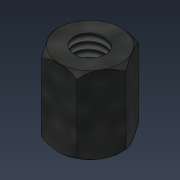
# Autodesk Inventor part: M2.5x5
Saved by Autodesk Inventor 2022.1 (Build 261234020, 234B)
## iProperties
Created: 2012-08-14
Part Number: M2.5x5
Material: Stahl
Document SubType Name: Modeling
Designer: rYan
Density: 7.85 g/cm^3
Mass: 3.36246 g
Surface Area: 5.74911 cm^2
Volume: 0.428339 cm^3
Appearance: Platte
Author: rYan
Autodesk Inventor part; units mm, degrees
ref_plane "YZ Plane" through (0, 0, 0) normal (1, 0, 0) x (0, 1, 0)
ref_plane "XZ Plane" through (0, 0, 0) normal (0, 1, 0) x (-1, 0, 0)
ref_plane "XY Plane" through (0, 0, 0) normal (0, 0, 1) x (1, 0, 0)
sketch "Skizze1" plane through (0, 0, 0) normal (0, 0, 1) x (1, 0, 0)
  line L0 (2.3094, 0) -> (1.1547, -2)
  line L1 (1.1547, -2) -> (-1.1547, -2)
  line L2 (-1.1547, -2) -> (-2.3094, 0)
  line L3 (-2.3094, 0) -> (-1.1547, 2)
  line L4 (-1.1547, 2) -> (1.1547, 2)
  line L5 (1.1547, 2) -> (2.3094, 0)
  point P0 (0, 0)
  point P1 (0, 0)
  dimension "SW" = 4
  constraints: 12 end point, 1 coincident, 13 other
  measures "SW" distance between parallel lines of L1 L4
extrude "Extrusion1" add sketch "Skizze1" along normal mid plane 5
sketch "Skizze2" plane through (0, 0, 2.5) normal (0, 0, 1) x (1, 0, 0)
  point P0 (0, 0)
  point P1 (0, 0)
  constraints: 1 coincident
hole "Bohrung1" at (0, 0, 2.5) direction (0, 0, -1) diameter 2.013 end through all thread size "M2.5x0.45" class "6H" standard "ISO Metric profile"
sketch "Innenradius" plane through (0, 0, 2.5) normal (0, 0, 1) x (1, 0, 0)
  circle A0 centre (0, 0) radius 2
  line L0 (2.3094, 0) -> (1.1547, 2) projected
  constraints: 1 centre point, 1 coincident, 1 tangent
sketch "Skizze7" plane through (0, 0, 0) normal (0, 1, 0) x (-1, 0, 0)
  line L0 (-1.0065, 2.5) -> (1.0065, 2.5) projected
  line L1 (-1.1547, 2.5) -> (-2.3094, 2.5) projected
  line L2 (-2.3094, 2.5) -> (-1.1547, 2.5) projected
  line L3 (-1.1547, 2.5) -> (1.1547, 2.5) projected
  line L4 (1.1547, 2.5) -> (2.3094, 2.5) projected
  line L5 (2.3094, 2.5) -> (1.1547, 2.5) projected
  line L6 (1.1547, 2.5) -> (-1.1547, 2.5) projected
  line L7 (1.0065, -2.5) -> (-1.0065, -2.5) projected
  line L8 (-2.3094, -2.5) -> (-1.1547, -2.5) projected
  line L9 (-1.1547, -2.5) -> (1.1547, -2.5) projected
  line L10 (1.1547, -2.5) -> (2.3094, -2.5) projected
  line L11 (2.3094, -2.5) -> (1.1547, -2.5) projected
  line L12 (1.1547, -2.5) -> (-1.1547, -2.5) projected
  line L13 (-1.1547, -2.5) -> (-2.3094, -2.5) projected
  line L14 (0, -4.2) -> (0, 4.2) projected
  line L15 (0, 2.5) -> (0, -2.5)
  line L16 (2, 2.5) -> (-2, 2.5) projected
  line L17 (2, 2.5) -> (2.3094, 2.5)
  line L18 (2.3094, 2.1906) -> (2, 2.5)
  line L19 (2.3094, 2.5) -> (2.3094, 2.1906)
  point P0 (0, 0)
  dimension "d16" = 45
  constraints: 8 end point, 2 midpoint, 2 point on line, 1 collinear, 1 perpendicular
  measures "d16" angle of L4 L18
revolve "Umdrehung1" cut sketch "Skizze7" angle 360 about axis through (0, 0, 0) along (0, 0, 1)
mirror "Spiegeln1" about plane through (0, 0, 0) normal (0, 0, 1) of "Umdrehung1"
